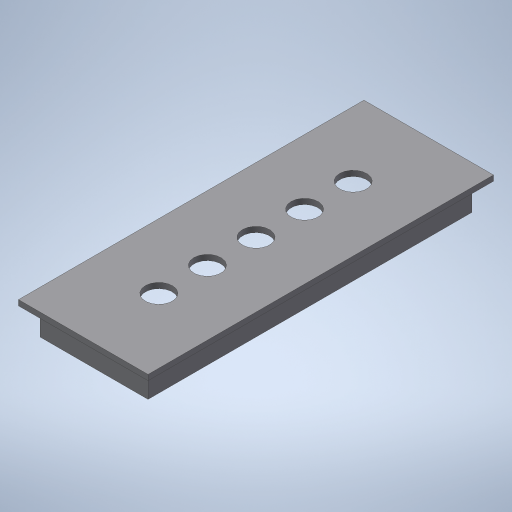
# Autodesk Inventor part: Parte 2.2 final
Saved by Autodesk Inventor 2023.1 (Build 271208000, 208)
## iProperties
Created: 2022-10-20
Part Number: Parte 2.2 final
Material: Generic
Document SubType Name: Modeling
Designer: User
Density: 1 g/cm^3
Appearance: Default
Author: User
Autodesk Inventor part; units mm, degrees
ref_plane "YZ Plane" through (0, 0, 0) normal (1, 0, 0) x (0, 1, 0)
ref_plane "XZ Plane" through (0, 0, 0) normal (0, 1, 0) x (-1, 0, 0)
ref_plane "XY Plane" through (0, 0, 0) normal (0, 0, 1) x (1, 0, 0)
sketch "Sketch1" plane through (0, 0, 0) normal (0, 1, 0) x (-1, 0, 0)
  line L0 (0, 0) -> (24, 0)
  line L1 (24, 0) -> (24, 64)
  line L2 (24, 64) -> (0, 64)
  line L3 (0, 64) -> (0, 0)
  dimension "d0" = 24
  dimension "d1" = 64
  constraints: 8 end point, 2 parallel, 1 horizontal, 1 perpendicular
  measures "d0" distance of L2.end L1.end
  measures "d1" distance of L1.end L0.end
extrude "Extrusion1" add sketch "Sketch1" along normal blind 1
sketch "Sketch2" plane through (0, 0, 0) normal (0, -1, 0) x (1, 0, 0)
  line L0 (-24, 0) -> (-24, 64) projected
  line L1 (0, 0) -> (-24, 0) projected
  line L2 (0, 64) -> (0, 0) projected
  line L3 (-24, 64) -> (0, 64) projected
  line L4 (-2, 2) -> (-22, 2)
  line L5 (-22, 2) -> (-22, 62)
  line L6 (-22, 62) -> (-2, 62)
  line L7 (-2, 62) -> (-2, 2)
  line L8 (-4, 4) -> (-20, 4)
  line L9 (-20, 4) -> (-20, 60)
  line L10 (-20, 60) -> (-4, 60)
  line L11 (-4, 60) -> (-4, 4)
  dimension "d4" = 2
  dimension "d5" = 2
  constraints: 16 end point, 6 other
  measures "d4" distance between parallel lines of L2 L7
  measures "d5" distance between parallel lines of L7 L11
extrude "Extrusion2" add sketch "Sketch2" along normal blind 5 contours L4 L5 L6 L7
sketch "Sketch3" plane through (0, 0, 0) normal (0, -1, 0) x (1, 0, 0)
  line L0 (-4, 4) -> (-4, 60) projected
  line L1 (-4, 60) -> (-20, 60) projected
  line L2 (-20, 60) -> (-20, 4) projected
  line L3 (-20, 4) -> (-4, 4) projected
  line L4 (-4, 4) -> (-20, 4) construction
  line L5 (-12, 4) -> (-12, 60) construction
  line L6 (-4, 60) -> (-20, 60) construction
  line L7 (-12, 4) -> (-12, 5) construction
  line L8 (-12, 60) -> (-12, 59) construction
  line L9 (-12, 59) -> (-12, 50) construction
  line L10 (-12, 50) -> (-12, 41) construction
  line L11 (-12, 41) -> (-12, 32) construction
  line L12 (-12, 32) -> (-12, 23) construction
  line L13 (-12, 23) -> (-12, 14) construction
  circle A0 centre (-12, 50) radius 2.5
  circle A1 centre (-12, 41) radius 2.5
  circle A2 centre (-12, 32) radius 2.5
  circle A3 centre (-12, 23) radius 2.5
  circle A4 centre (-12, 14) radius 2.5
  point P0 (0, 0)
  dimension "d8" = 1
  dimension "d9" = 1
  dimension "d10" = 9
  dimension "d11" = 9
  dimension "d12" = 9
  dimension "d13" = 9
  dimension "d14" = 9
  dimension "d15" = 5
  dimension "d16" = 5
  dimension "d17" = 5
  dimension "d18" = 5
  dimension "d19" = 5
  constraints: 14 end point, 10 coincident, 5 centre point, 2 midpoint, 10 other
  measures "d8" distance of L7.start L7.end
  measures "d9" distance of L8.start L8.end
  measures "d10" distance of L8.end L9.end
  measures "d11" distance of L9.end L10.end
  measures "d12" distance of L10.end L11.end
  measures "d13" distance of L11.end L12.end
  measures "d14" distance of L12.end L13.end
  measures "d15" diameter of A0
  measures "d16" diameter of A1
  measures "d17" diameter of A2
  measures "d18" diameter of A3
  measures "d19" diameter of A4
extrude "Extrusion3" cut sketch "Sketch3" against normal blind 2 contours A0 | A1 | A2 | A3 | A4
body "Solid1"
